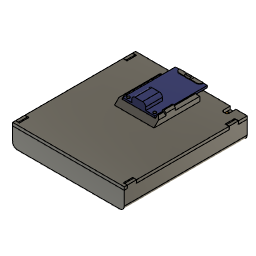
battery-case (Autodesk Fusion 360 design; units mm, degrees)
Autodesk Fusion 360 part; units mm, degrees
sketch "Battery-sketch" plane through (0, 0, 0) normal (0, 0, 1) x (1, 0, 0)
  line L0 (56, 62) -> (0, 62)
  line L1 (0, 62) -> (0, 0)
  line L2 (0, 0) -> (56, 0)
  line L3 (56, 0) -> (56, 62)
  line L4 (0, -75) -> (0, 75) construction
  line L5 (-75, 0) -> (75, 0) construction
  dimension "d1" = 56
  dimension "d2" = 62
  constraint horizontal L0
  constraint vertical L1
  constraint horizontal L2
  constraint vertical L3
  constraint perpendicular L0 L4
  constraint horizontal L5
  constraint coincident L1.end L2.start
  measures "d1" distance of L0.start L0.end
  measures "d2" distance of L0.start L2.end
extrude "Extrude1" add sketch "Battery-sketch" along normal blind 8.1 makes body 1
fillet "Fillet1" radius 3 4 edges at (56, 31, 8.1) (56, 31, 0) (0, 31, 8.1) (0, 31, 0) on bodies 1
sketch "Charger-sketch" plane through (0, 0, 0) normal (0, 0, 1) x (1, 0, 0)
  line L0 (17, 0) -> (17, 28)
  line L1 (0, 28) -> (0, 0)
  line L2 (4.825, 8.94) -> (12.175, 8.94)
  line L3 (12.175, 8.94) -> (12.175, 0)
  line L4 (4.825, 0) -> (4.825, 8.94)
  line L5 (0, 0) -> (4.825, 0)
  line L6 (12.175, 0) -> (17, 0)
  line L7 (4.825, 0) -> (12.175, 0)
  line L8 (4, 26) -> (13, 26)
  line L9 (2, 29) -> (2, 29)
  line L10 (17, 28) -> (15, 28)
  line L11 (2, 28) -> (0, 28)
  arc A0 (13, 26) -> (15, 28) centre (13, 28) ccw
  arc A1 (2, 28) -> (4, 26) centre (4, 28) ccw
  circle A2 centre (15.5, 1.5) radius 0.75
  circle A3 centre (1.5, 1.5) radius 0.75
  dimension "d7" = 17
  dimension "d8" = 28
  dimension "d9" = 7.35
  dimension "d10" = 8.94
  dimension "d11" = 2
  dimension "d13" = 2
  dimension "d16" = 2
  dimension "d117" = 2
  dimension "d118" = 1.5
  dimension "d119" = 1.5
  dimension "d120" = 1.5
  dimension "d121" = 1.5
  dimension "d122" = 1.5
  dimension "d123" = 1.5
  constraint horizontal L5
  constraint vertical L0
  constraint horizontal L10
  constraint vertical L1
  constraint coincident L1.end L5.start
  constraint horizontal L2
  constraint vertical L3
  constraint vertical L4
  constraint coincident L3.end L5
  constraint collinear L5 L6
  constraint equal L5 L6
  constraint perpendicular L1 L8
  constraint coincident L11.start L10
  constraint collinear L10 L11
  constraint equal L10 L11
  constraint tangent L8 A0
  constraint tangent L8 A1
  constraint equal A0 A1
  constraint coincident L10.end A0.end
  measures "d7" distance of L1.end L0.start
  measures "d8" distance of L1.end L1.start
  measures "d9" distance of L2.start L2.end
  measures "d10" distance of L2.start L4.start
  measures "d11" distance of L8 L11
  measures "d13" radius of A0
  measures "d16" horizontal distance of L11.start L8.start
  measures "d117" distance of L1.start L11.start
  measures "d118" diameter of A2
  measures "d119" distance of L6 A2.centre
  measures "d120" distance of L0 A2.centre
  measures "d121" diameter of A3
  measures "d122" distance of L1 A3.centre
  measures "d123" distance of L5 A3.centre
extrude "Extrude2" add sketch "Charger-sketch" along normal blind 1 separate body contours L0 L1 L2 L3 L4 L5 L6 L8 L10 L11 A0 A1 makes body 2
extrude "Extrude3" add sketch "Charger-sketch" along normal blind 4.3 contours L2 L3 L4 L7 bodies 2
fillet "Fillet2" radius 1.65 2 edges at (12.175, 4.47, 4.3) (4.825, 4.47, 4.3) on bodies 2
move_body "Move1" bodies 2 to x (1, 0, 0) y (0, 1, 0) z (0, 0, 1) at (-24, 0, 0)
sketch "Case-bottom-sketch" plane through (0, 0, 0) normal (0, 0, 1) x (1, 0, 0)
  line L0 (0, 62.2) -> (57.2, 62.2)
  line L1 (56.2, 59.2) -> (56.2, 0)
  line L2 (56.2, 0) -> (0, 0)
  line L3 (0, 0) -> (0, 62.2)
  line L4 (-1.6, 63.8) -> (57.8, 63.8)
  line L5 (57.8, 63.8) -> (57.8, -1.6)
  line L6 (57.8, -1.6) -> (-1.6, -1.6)
  line L7 (-1.6, -1.6) -> (-1.6, 63.8)
  line L8 (0, 4.9) -> (-1.6, 4.9)
  line L9 (0, 4.9) -> (0.5, 4.9)
  line L10 (0.5, 4.9) -> (0.5, 0.1)
  line L11 (57.8, 4.9) -> (56.2, 4.9)
  line L12 (56.2, 4.9) -> (55.7, 4.9)
  line L13 (55.7, 4.9) -> (55.7, 0.1)
  line L14 (0, 57.3) -> (-1.6, 57.3)
  line L15 (0, 57.3) -> (0.5, 57.3)
  line L16 (0.5, 57.3) -> (0.5, 62.1)
  line L17 (57.8, 54.3) -> (56.2, 54.3)
  line L18 (56.2, 54.3) -> (55.7, 54.3)
  line L19 (55.7, 54.3) -> (55.7, 59.1)
  line L20 (57.2, 62.2) -> (57.8, 62.2)
  line L21 (5.1, 57.1) -> (51.1, 57.1)
  line L22 (51.1, 57.1) -> (51.1, 5.1)
  line L23 (51.1, 5.1) -> (5.1, 5.1)
  line L24 (5.1, 5.1) -> (5.1, 57.1)
  line L25 (-1.6, 0.1) -> (0, 0.1)
  line L26 (0, 62.1) -> (-1.6, 62.1)
  line L27 (57.8, 59.1) -> (56.2, 59.1)
  line L28 (0, 62.1) -> (0.5, 62.1)
  line L29 (0.5, 0.1) -> (0, 0.1)
  line L30 (57.8, 0.1) -> (55.7, 0.1)
  line L31 (56.2, 59.1) -> (55.7, 59.1)
  line L32 (56.2, 59.2) -> (56.2, 62.2)
  dimension "d23" = 1.6
  dimension "d24" = 1.6
  dimension "d25" = 1.6
  dimension "d26" = 1.6
  dimension "d27" = 56.2
  dimension "d28" = 62.2
  dimension "d31" = 0.5
  dimension "d32" = 0.5
  dimension "d34" = 0.5
  dimension "d36" = 0.5
  dimension "d54" = 5.1
  dimension "d55" = 5.1
  dimension "d56" = 5.1
  dimension "d57" = 5.1
  dimension "d125" = 0.1
  dimension "d126" = 4.8
  dimension "d127" = 0.1
  dimension "d128" = 4.8
  dimension "d130" = 4.8
  dimension "d131" = 0.1
  dimension "d132" = 4.8
  dimension "d147" = 3.1
  constraint horizontal L0
  constraint vertical L1
  constraint horizontal L2
  constraint vertical L3
  constraint horizontal L4
  constraint vertical L5
  constraint horizontal L6
  constraint vertical L7
  constraint coincident L1.end L2.start
  constraint coincident L0.start L3.end
  constraint coincident L2.end L3.start
  constraint coincident L3 L8.start
  constraint perpendicular L7 L8
  constraint perpendicular L3 L9
  constraint perpendicular L2 L10
  constraint coincident L1 L11.end
  constraint perpendicular L1 L11
  constraint perpendicular L1 L12
  constraint perpendicular L2 L13
  constraint coincident L3 L14.start
  constraint perpendicular L7 L14
  constraint perpendicular L3 L15
  constraint perpendicular L0 L16
  constraint coincident L1 L17.end
  constraint perpendicular L1 L17
  constraint perpendicular L1 L18
  constraint perpendicular L0 L19
  constraint coincident L5 L20.end
  constraint perpendicular L5 L20
  constraint perpendicular L3 L21
  constraint perpendicular L21 L22
  constraint perpendicular L22 L23
  constraint perpendicular L21 L24
  constraint coincident L7 L14.end
  constraint coincident L7 L8.end
  constraint coincident L5 L11.start
  constraint coincident L5 L17.start
  constraint coincident L7 L25.start
  constraint coincident L3 L25.end
  constraint perpendicular L3 L25
  constraint coincident L3 L26.start
  constraint coincident L7 L26.end
  constraint perpendicular L7 L26
  constraint coincident L5 L27.start
  constraint coincident L1 L27.end
  constraint perpendicular L1 L27
  constraint perpendicular L16 L28
  constraint collinear L25 L29
  constraint coincident L5 L30.start
  constraint perpendicular L13 L30
  constraint perpendicular L19 L31
  constraint coincident L0 L32.end
  constraint perpendicular L0 L32
  measures "d23" distance of L3 L7
  measures "d24" distance of L1 L5
  measures "d25" distance of L2 L6
  measures "d26" distance of L0 L4
  measures "d27" distance of L2.end L1.end
  measures "d28" distance of L0 L2
  measures "d31" distance of L3 L10
  measures "d32" distance of L11.end L12.end
  measures "d34" distance of L14.start L15.end
  measures "d36" distance of L17.end L18.end
  measures "d54" distance of L0 L21
  measures "d55" distance of L2 L23
  measures "d56" distance of L1 L22
  measures "d57" distance of L3 L24
  measures "d125" distance of L2.end L25
  measures "d126" distance of L8 L25
  measures "d127" distance of L0.start L26
  measures "d128" distance of L14 L26
  measures "d130" distance of L17 L27
  measures "d131" distance of L1.end L30
  measures "d132" distance of L11 L30
  measures "d147" distance of L0 L27
extrude "Extrude4" add sketch "Case-bottom-sketch" along normal blind 1.6 separate body contours L0 L1 L2 L3 L9 L10 L12 L13 L15 L16 L18 L19 L28 L29 L30 L31 L32 | L3 L15 L16 L28 | L1 L18 L19 L31 | L3 L9 L10 L29 | L1 L12 L13 L30 makes body 3
extrude "Extrude5" add sketch "Case-bottom-sketch" along normal blind 9.8 contours L0 L3 L4 L5 L7 L20 L26 | L0 L1 L5 L20 L27 L32 | L3 L7 L8 L14 | L1 L5 L11 L17 | L1 L2 L3 L5 L6 L7 L25 L30 bodies 3
extrude "Extrude6" add sketch "Case-bottom-sketch" along normal blind 11.4 contours L3 L7 L14 L26 | L1 L5 L17 L27 | L3 L7 L8 L25 | L1 L5 L11 L30 bodies 3
extrude "Extrude7" add sketch "Case-bottom-sketch" along normal blind 11.4 and the other way blind -10.6 contours L3 L15 L16 L28 | L1 L18 L19 L31 | L3 L9 L10 L29 | L1 L12 L13 L30 bodies 3
chamfer "Chamfer1" distance 0.6 angle 45 4 edges at (0.5, 2.5, 11.4) (0.5, 59.7, 11.4) (55.7, 2.5, 11.4) (55.7, 56.7, 11.4) on bodies 3
fillet "Fillet3" radius 2.5 4 edges at (-1.6, 31.1, 0) (0, 31.1, 1.6) (56.2, 31.1, 1.6) (57.8, 31.1, 0) on bodies 3
fillet "Fillet4" radius 2.5 4 edges at (5.1, 57.1, 0.8) (51.1, 57.1, 0.8) (51.1, 5.1, 0.8) (5.1, 5.1, 0.8) on bodies 3
move_body "Move2" bodies 1 to x (1, 0, 0) y (0, 1, 0) z (0, 0, 1) at (0, 0, 1.6)
move_body "Move3" bodies 1 to x (1, 0, 0) y (0, 1, 0) z (0, 0, 1) at (0, 0.1, 0)
sketch "Case-top-sketch" plane through (0, 0, 0) normal (0, 0, 1) x (1, 0, 0)
  line L0 (-1.6, -1.6) -> (57.8, -1.6)
  line L1 (-1.6, 57.2) -> (0, 57.2)
  line L2 (0, 57.2) -> (0, 62.2)
  line L3 (0, 62.2) -> (-1.6, 62.2)
  line L4 (-1.6, 5) -> (0, 5)
  line L5 (0, 5) -> (0, 0)
  line L6 (0, 0) -> (-1.6, 0)
  line L7 (57.8, 0) -> (56.2, 0)
  line L8 (56.2, 0) -> (56.2, 5)
  line L9 (56.2, 5) -> (57.8, 5)
  line L10 (56.2, 54.2) -> (57.8, 54.2)
  line L11 (56.2, 59.2) -> (56.2, 54.2)
  line L12 (56.2, 59.2) -> (57.8, 59.2)
  line L13 (-1.6, 63.8) -> (-1.6, 62.2)
  line L14 (-1.6, 57.2) -> (-1.6, 5)
  line L15 (-1.6, 0) -> (-1.6, -1.6)
  line L16 (57.8, -1.6) -> (57.8, 0)
  line L17 (57.8, 5) -> (57.8, 54.2)
  line L18 (57.8, 59.2) -> (57.8, 63.8)
  line L19 (0.5, 57.2) -> (0, 57.2)
  line L20 (56.2, 59.2) -> (55.7, 59.2)
  line L21 (55.7, 59.2) -> (55.7, 54.2)
  line L22 (55.7, 54.2) -> (56.2, 54.2)
  line L23 (55.7, 5) -> (56.2, 5)
  line L24 (0, 0) -> (0.5, 0)
  line L25 (0.5, 0) -> (0.5, 5)
  line L26 (0.5, 5) -> (0, 5)
  line L27 (57.8, 63.8) -> (34.5, 63.8)
  line L28 (21.7, 63.8) -> (-1.6, 63.8)
  line L29 (21.7, 63.8) -> (34.5, 63.8)
  arc A0 (32.55, 61.85) -> (34.5, 63.8) centre (32.55, 63.8) ccw
  arc A1 (21.7, 63.8) -> (23.65, 61.85) centre (23.65, 63.8) ccw
  line L30 (26.6, 62.95) -> (29.6, 62.95)
  line L31 (26.6, 62.95) -> (26.6, 61.85)
  line L32 (29.6, 62.95) -> (29.6, 61.85)
  line L33 (23.65, 61.85) -> (26.6, 61.85)
  line L34 (29.6, 61.85) -> (32.55, 61.85)
  line L35 (26.6, 61.85) -> (29.6, 61.85)
  line L36 (26.6, 61.85) -> (26.6, 61.35)
  line L37 (26.6, 61.35) -> (29.6, 61.35)
  line L38 (29.6, 61.35) -> (29.6, 61.85)
  line L39 (19.2, 57.85) -> (37, 57.85)
  line L40 (19.2, 57.85) -> (19.2, 35.8)
  line L41 (19.2, 35.8) -> (37, 35.8)
  line L42 (37, 57.85) -> (37, 35.8)
  line L43 (19.2, 57.85) -> (17.6, 57.85)
  line L44 (17.6, 57.85) -> (17.6, 35.8)
  line L45 (19.2, 35.8) -> (17.6, 35.8)
  line L46 (37, 57.85) -> (38.6, 57.85)
  line L47 (38.6, 57.85) -> (38.6, 35.8)
  line L48 (37, 35.8) -> (38.6, 35.8)
  line L49 (37, 39.8) -> (38.1, 39.8)
  line L50 (38.1, 39.8) -> (38.1, 44.8)
  line L51 (38.1, 44.8) -> (37, 44.8)
  line L52 (37, 44.8) -> (36.5, 44.8)
  line L53 (36.5, 44.8) -> (36.5, 39.8084)
  line L54 (37, 39.8) -> (36.5, 39.8084)
  circle A2 centre (21.05, 37.3) radius 0.7
  circle A3 centre (35.15, 37.3) radius 0.7
  line L55 (0, 62.2) -> (0.5, 62.2)
  line L56 (0.5, 62.2) -> (0.5, 57.2)
  line L57 (56.2, 0) -> (55.7, 0)
  line L58 (55.7, 0) -> (55.7, 5)
  line L59 (48.8, 63.8) -> (48.8, 59.2)
  line L60 (48.8, 59.2) -> (51.8, 59.2)
  line L61 (51.8, 59.2) -> (51.8, 63.8)
  point P0 (-1.6, 63.8)
  point P1 (-1.6, -1.6)
  point P2 (57.8, -1.6)
  point P3 (57.8, 63.8)
  point P4 (0, 62.2)
  point P5 (56.2, 0)
  point P6 (21.4907, 62.85)
  point P7 (34.6907, 61.85)
  dimension "d64" = 1.95
  dimension "d65" = 1.95
  dimension "d66" = 1.95
  dimension "d67" = 12.8
  dimension "d68" = 1.1
  dimension "d69" = 3
  dimension "d70" = 0.5
  dimension "d71" = 17.8
  dimension "d72" = 2.5
  dimension "d73" = 4
  dimension "d74" = 28
  dimension "d75" = 1.6
  dimension "d76" = 1.6
  dimension "d77" = 5
  dimension "d78" = 1.1
  dimension "d79" = 0.5
  dimension "d80" = 4
  dimension "d81" = 1.4
  dimension "d82" = 1.85
  dimension "d83" = 1.5
  dimension "d84" = 1.4
  dimension "d85" = 1.5
  dimension "d86" = 1.85
  dimension "d124" = 2.5
  dimension "d134" = 1.6
  dimension "d135" = 5
  dimension "d136" = 0.5
  dimension "d138" = 1.6
  dimension "d139" = 5
  dimension "d140" = 1.6
  dimension "d141" = 0.5
  dimension "d142" = 5
  dimension "d143" = 0.5
  dimension "d144" = 5
  dimension "d145" = 1.6
  dimension "d146" = 0.5
  dimension "d149" = 6
  dimension "d151" = 3
  dimension "d154" = 4.6
  dimension "d155" = 4.6
  constraint coincident P0 L13.start
  constraint coincident P1 L0.start
  constraint coincident P2 L0.end
  constraint coincident P3 L18.end
  constraint coincident L1.start L13
  constraint perpendicular L1 L13
  constraint perpendicular L3 L13
  constraint coincident L4.start L13
  constraint perpendicular L4 L13
  constraint coincident L5.end L6.start
  constraint coincident L6.end L13
  constraint perpendicular L6 L13
  constraint coincident P5 L7.end
  constraint perpendicular L7 L16
  constraint coincident L9.end L16
  constraint perpendicular L9 L16
  constraint coincident L10.end L16
  constraint perpendicular L10 L16
  constraint coincident L12.end L18.start
  constraint collinear L13 L14
  constraint collinear L14 L15
  constraint collinear L16 L17
  constraint collinear L17 L18
  constraint perpendicular L5 L24
  constraint perpendicular L6 L25
  constraint horizontal L33
  constraint coincident L28.start L27
  constraint collinear L27 L28
  constraint equal L27 L28
  constraint coincident P7 L33
  constraint tangent A0 L33
  constraint tangent A1 L33
  constraint coincident L27 L29.end
  constraint coincident L27.end L29.end
  constraint coincident L29 L28.start
  constraint coincident L28.start L29.start
  constraint parallel L30 L33
  constraint perpendicular L31 L33
  constraint coincident L32.end L33
  constraint perpendicular L32 L33
  constraint collinear L33 L34
  constraint equal L33 L34
  constraint perpendicular L33 L36
  constraint perpendicular L36 L37
  constraint perpendicular L34 L38
  constraint parallel L28 L39
  constraint perpendicular L39 L40
  constraint perpendicular L40 L41
  constraint perpendicular L41 L42
  constraint perpendicular L40 L43
  constraint perpendicular L43 L44
  constraint perpendicular L44 L45
  constraint perpendicular L42 L46
  constraint perpendicular L46 L47
  constraint perpendicular L47 L48
  constraint coincident L42 L49.start
  constraint perpendicular L42 L49
  constraint perpendicular L49 L50
  constraint coincident L42 L51.end
  constraint perpendicular L42 L51
  constraint perpendicular L42 L52
  constraint perpendicular L52 L53
  constraint perpendicular L2 L55
  constraint perpendicular L8 L57
  constraint collinear L1 L19
  constraint coincident L19.start L56.end
  constraint collinear L4 L26
  constraint coincident L23.start L58.end
  constraint collinear L9 L23
  constraint perpendicular L8 L9
  constraint collinear L12 L20
  constraint collinear L10 L22
  constraint perpendicular L27 L59
  constraint perpendicular L59 L60
  constraint perpendicular L60 L61
  constraint coincident L27 L59.start
  constraint coincident L27 L61.end
  measures "d64" radius of A0
  measures "d65" radius of A1
  measures "d66" distance of L29 L33
  measures "d67" distance of L27.end L28.start
  measures "d68" distance of L30 L33
  measures "d69" distance of L30.start L30.end
  measures "d70" distance of L32.end L37.end
  measures "d71" distance of L39.start L39.end
  measures "d72" horizontal distance of L27.end L39.end
  measures "d73" distance of L34 L39
  measures "d74" distance of L28 L41
  measures "d75" distance of L40 L44
  measures "d76" distance of L42 L47
  measures "d77" distance of L49.end L50.end
  measures "d78" distance of L42 L50
  measures "d79" distance of L51.end L52.end
  measures "d80" distance of L48 L49
  measures "d81" diameter of A2
  measures "d82" distance of L40 A2.centre
  measures "d83" distance of L41 A2.centre
  measures "d84" diameter of A3
  measures "d85" distance of L41 A3.centre
  measures "d86" distance of L42 A3.centre
  measures "d124" horizontal distance of L28.start L39.start
  measures "d134" distance of L3 L28
  measures "d135" distance of L1 L3
  measures "d136" distance of L2 L56
  measures "d138" distance of L2 L13
  measures "d139" distance of L4 L6
  measures "d140" distance of L5 L14
  measures "d141" distance of L5 L25
  measures "d142" distance of L7 L9
  measures "d143" distance of L8 L58
  measures "d144" distance of L10 L12
  measures "d145" distance of L11 L18
  measures "d146" distance of L11 L21
  measures "d149" distance of L18 L61
  measures "d151" distance of L59 L61
  measures "d154" distance of L27 L60
  measures "d155" distance of P3 L12.end
extrude "Extrude8" add sketch "Case-top-sketch" along normal blind 11.4 and the other way blind -9.8 separate body contours L0 L1 L3 L4 L6 L7 L9 L10 L12 L13 L14 L15 L16 L17 L18 L19 L20 L21 L22 L23 L24 L25 L26 L27 L28 A0 A1 L33 L34 L36 L37 L38 L55 L56 L57 L58 L59 L60 L61 | L35 L36 L37 L38 makes body 4
extrude "Extrude9" add sketch "Case-top-sketch" along normal blind 10.6 and the other way blind -9.8 contours L5 L24 L25 L26 | L8 L23 L57 L58 | L2 L19 L55 L56 | L11 L20 L21 L22 bodies 4
extrude "Extrude10" add sketch "Case-top-sketch" along normal blind 13.8 and the other way blind -9.8 contours L39 L40 L41 L42 L52 L53 L54 | L42 L52 L53 L54 bodies 4
extrude "Extrude11" add sketch "Case-top-sketch" along normal blind 15 and the other way blind -9.8 contours L29 A0 A1 L30 L31 L32 L33 L34 | L40 L43 L44 L45 | L42 L46 L47 L48 L49 L50 L51 | A2 | A3 bodies 4
extrude "Extrude12" add sketch "Case-top-sketch" along normal blind 16 and the other way blind -9.8 contours L30 L31 L32 L35 | L42 L49 L50 L51 bodies 4
extrude "Extrude13" add sketch "Case-top-sketch" along normal blind 16 and the other way blind -15.2 contours L35 L36 L37 L38 | L42 L52 L53 L54 bodies 4 3
chamfer "Chamfer2" distance 0.6 angle 45 2 edges at (28.1, 61.35, 16) (36.5, 42.3042, 16) on bodies 4
chamfer "Chamfer3" distance 0.8 angle 45 1 edges at (28.1, 62.95, 15) on bodies 4
chamfer "Chamfer4" distance 0.5 angle 45 1 edges at (38.1, 42.3, 15) on bodies 4
chamfer "Chamfer5" distance 0.5 angle 45 1 edges at (38.1, 42.3, 16) on bodies 4
chamfer "Chamfer6" distance 1.2 angle 45 8 edges at (17.6, 46.825, 15) (38.6, 37.8, 15) (38.6, 51.325, 15) (28.1, 57.85, 13.8) (37.8, 57.85, 15) (18.4, 57.85, 15) (18.4, 35.8, 15) (37.8, 35.8, 15) on bodies 4
chamfer "Chamfer7" distance 2.4 angle 45 1 edges at (28.1, 35.8, 11.4) on bodies 4
move_body "Move4" bodies 2 to x (1, 0, 0) y (0, 1, 0) z (0, 0, 1) at (43.6, 35.8, 13.4)
fillet "Fillet5" radius 1 2 edges at (48.8, 59.2, 10.6) (51.8, 59.2, 10.6) on bodies 4
move_body "Move5" bodies 2 to x (1, 0, 0) y (0, 1, 0) z (0, 0, 1) at (0, 0, 0.4)
chamfer "Chamfer8" distance 0.2 angle 45 1 edges at (28.1, 62.95, 16) on bodies 4
sketch "Sketch5" plane through (-1.6, 0, 0) normal (-1, 0, 0) x (0, -1, 0)
  line L0 (-63.8, 2.5) -> (1.6, 2.5)
  line L1 (1.6, 2.5) -> (1.6, 9.8)
  line L2 (1.6, 9.8) -> (-0.1, 9.8)
  line L3 (-0.1, 9.8) -> (-0.1, 11.4)
  line L4 (-0.1, 11.4) -> (-4.9, 11.4)
  line L5 (-4.9, 11.4) -> (-4.9, 9.8)
  line L6 (-4.9, 9.8) -> (-57.3, 9.8)
  line L7 (-57.3, 9.8) -> (-57.3, 11.4)
  line L8 (-57.3, 11.4) -> (-62.1, 11.4)
  line L9 (-62.1, 11.4) -> (-62.1, 9.8)
  line L10 (-62.1, 9.8) -> (-63.8, 9.8)
  line L11 (-63.8, 9.8) -> (-63.8, 2.5)
  line L12 (-46.1, 9.8) -> (-16.1, 9.8)
  line L13 (-16.1, 9.8) -> (-16.1, -4.5)
  line L14 (-16.1, -4.5) -> (-46.1, -4.5)
  line L15 (-46.1, -4.5) -> (-46.1, 9.8)
  line L16 (-63.8, 0) -> (1.6, 0)
  line L17 (-44.1, 0) -> (-18.1, 0)
  line L18 (-18.1, 0) -> (-18.1, -2.5)
  line L19 (-18.1, -2.5) -> (-44.1, -2.5)
  line L20 (-44.1, -2.5) -> (-44.1, 0)
  dimension "d157" = 30
  dimension "d158" = 4.5
  dimension "d159" = 17.7
  dimension "d160" = 17.7
  dimension "d161" = 2
  dimension "d162" = 2
  dimension "d163" = 2
  constraint horizontal L12
  constraint vertical L13
  constraint horizontal L14
  constraint vertical L15
  constraint collinear L6 L12
  constraint horizontal L17
  constraint vertical L18
  constraint horizontal L19
  constraint vertical L20
  constraint collinear L16 L17
  measures "d157" distance of L12.start L12.end
  measures "d158" distance of L14 L16
  measures "d159" distance of L1 L13
  measures "d160" distance of L11 L15
  measures "d161" distance of L14 L19
  measures "d162" distance of L15 L20
  measures "d163" distance of L13 L18
extrude "Extrude14" add sketch "Sketch5" along normal blind 2 separate body contours L0 L6 L12 L13 L15 | L0 L13 L15 L16 L17 | L13 L14 L15 L16 L18 L19 L20 makes body 5
sketch "Sketch6" plane through (0, 63.8, 0) normal (0, 1, 0) x (-1, 0, 0)
  arc A0 (-57.8, 2.5) -> (-55.3, 0) centre (-55.3, 2.5) ccw
  line L0 (-55.3, 0) -> (-0.9, 0)
  arc A1 (-0.9, 0) -> (1.6, 2.5) centre (-0.9, 2.5) ccw
  line L1 (1.6, 2.5) -> (1.6, 9.8)
  line L2 (1.6, 9.8) -> (-57.8, 9.8)
  line L3 (-57.8, 9.8) -> (-57.8, 2.5)
  arc A2 (-0.9, 0) -> (1.6, 2.5) centre (-0.9, 2.5) ccw
  line L4 (-0.9, 0) -> (1.6, 0)
  line L5 (1.6, -4.5) -> (1.6, 9.8)
  line L6 (1.6, 0) -> (1.6, 2.5)
  constraint coincident L0.end A1.start
  constraint tangent A2 L4
  constraint coincident L4.end L5
  constraint coincident A1.end L1.start
extrude "Extrude15" add sketch "Sketch6" along normal blind -47.7 and the other way blind 17.7 contours A1 A2 L4 L5 L6 bodies 5
chamfer "Chamfer9" distance 1.5 angle 45 2 edges at (-2.6, 16.1, -4.5) (-2.6, 46.1, -4.5) on bodies 5
chamfer "Chamfer10" distance 2 angle 45 1 edges at (-3.6, 31.1, 9.8) on bodies 5
chamfer "Chamfer11" distance 0.5 angle 45 4 edges at (-1.6, 31.1, -2.5) (-3.6, 31.1, -2.5) (-3.6, 31.1, -4.5) (-1.6, 31.1, -4.5) on bodies 5
chamfer "Chamfer12" distance 1.5 angle 45 1 edges at (0.9, 31.1, 0) on bodies 5
equation "d158 = 2.5 mm + 2 mm"
named bodies: "battery", "charger", "battery-case-top", "battery-case-bottom", "wristband"
